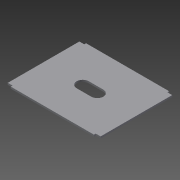
# Autodesk Inventor part: top_cover_sheet
Saved by Autodesk Inventor 2014 SP1 (Build 180222100, 222)
## iProperties
Created: 2014-02-23
Part Number: top_cover_sheet
Material: Wood (Birch)
Document SubType Name: Modeling
Designer: Chris
Density: 0.55 g/cm^3
Appearance: Birch - Natural Polished
Mass: 954.9 g
Surface Area: 3846.58 cm^2
Volume: 1736.18 cm^3
Author: Chris
Autodesk Inventor part; units mm, degrees
ref_plane "YZ Plane" through (0, 0, 0) normal (1, 0, 0) x (0, 1, 0)
ref_plane "XZ Plane" through (0, 0, 0) normal (0, 1, 0) x (-1, 0, 0)
ref_plane "XY Plane" through (0, 0, 0) normal (0, 0, 1) x (1, 0, 0)
sketch "Sketch1" plane through (0, 0, 0) normal (0, 0, 1) x (1, 0, 0)
  line L0 (0, 0) -> (485.775, 0)
  line L1 (485.775, 0) -> (485.775, 9.525)
  line L2 (485.775, 9.525) -> (0, 9.525)
  line L3 (0, 9.525) -> (0, 0)
  dimension "d0" = 485.775
  dimension "d1" = 9.525
  constraints: 8 end point, 2 parallel, 1 horizontal, 1 perpendicular
  measures "d0" distance of L1.end L2.end
  measures "d1" distance of L0.end L1.end
extrude "Extrusion1" add sketch "Sketch1" along normal blind 187.325
sketch "Sketch2" plane through (0, 0, 187.325) normal (0, 0, 1) x (1, 0, 0)
  line L0 (0, 0) -> (485.775, 0) projected
  line L1 (485.775, 0) -> (485.775, 9.525) projected
  line L2 (485.775, 9.525) -> (0, 9.525) projected
  line L3 (0, 9.525) -> (0, 0) projected
  line L4 (25.4, 9.525) -> (460.375, 9.525)
  line L5 (460.375, 9.525) -> (460.375, 0)
  line L6 (460.375, 0) -> (25.4, 0)
  line L7 (25.4, 0) -> (25.4, 9.525)
  dimension "d4" = 25.4
  dimension "d5" = 25.4
  constraints: 8 end point, 2 parallel, 2 point on line, 1 horizontal, 1 perpendicular
  measures "d4" distance between parallel lines of L3 L7
  measures "d5" distance between parallel lines of L1 L5
extrude "Extrusion2" add sketch "Sketch2" along normal blind 9.525 contours L7 L2 L5 L0
mirror "Mirror1" about plane through (242.8875, 4.7625, 0) normal (0, 0, -1)
sketch "Sketch3" plane through (25.4, 9.525, 196.85) normal (0, 1, 0) x (1, 0, 0)
  line L0 (-25.4, 384.175) -> (-25.4, 9.525) projected
  line L1 (0, 9.525) -> (-25.4, 9.525) projected
  line L2 (460.375, 384.175) -> (460.375, 9.525) projected
  line L3 (434.975, 393.7) -> (0, 393.7) projected
  line L4 (179.3875, 196.85) -> (255.5875, 196.85) construction
  line L5 (179.3875, 165.1) -> (255.5875, 165.1)
  line L6 (255.5875, 228.6) -> (179.3875, 228.6)
  arc A0 (179.3875, 228.6) -> (179.3875, 165.1) centre (179.3875, 196.85) ccw
  arc A1 (255.5875, 165.1) -> (255.5875, 228.6) centre (255.5875, 196.85) ccw
  point P0 (-25.4, 196.85)
  point P1 (217.4875, 196.85)
  dimension "d8" = 76.2
  dimension "d9" = 31.75
  dimension "d10" = 196.85
  dimension "d11" = 242.8875
  dimension "d12" = 242.8875
  constraints: 8 end point, 4 point on circle, 4 tangent, 2 centre point, 2 parallel, 1 midpoint
  measures "d8" distance of L6.start L6.end
  measures "d9" radius of A1
  measures "d10" distance between parallel lines of L3 L4
  measures "d11" distance from line of L0 point (217.488, 196.85)
  measures "d12" distance from line of L2 point (217.488, 196.85)
extrude "Extrusion3" cut sketch "Sketch3" against normal through all
equation "\"d11\" = d12"
body "Solid1"
